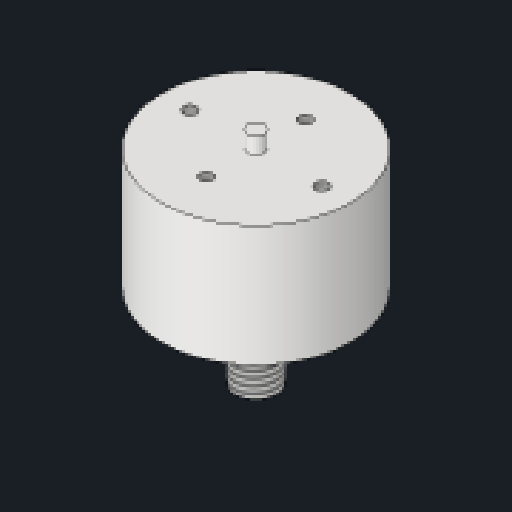
# Autodesk Inventor part: Emax 1806 2280kv
Saved by Autodesk Inventor 2023.2 (Build 272271030, 271C)
## iProperties
Created: 2024-02-18
Part Number: Emax 1806 2280kv
Material: Generic
Document SubType Name: Modeling
Designer: robpl
Density: 1 g/cm^3
Appearance: Default
Author: robpl
Autodesk Inventor part; units mm, degrees
ref_plane "YZ Plane" through (0, 0, 0) normal (1, 0, 0) x (0, 1, 0)
ref_plane "XZ Plane" through (0, 0, 0) normal (0, 1, 0) x (-1, 0, 0)
ref_plane "XY Plane" through (0, 0, 0) normal (0, 0, 1) x (1, 0, 0)
sketch "Sketch1" plane through (0, 0, 0) normal (0, 0, 1) x (1, 0, 0)
  line L0 (0, 0) -> (-11.5, 0)
  line L1 (-11.5, 0) -> (-11.5, -24.7)
  line L2 (-11.5, -24.7) -> (0, -24.7)
  line L3 (0, -24.7) -> (0, 0)
  line L4 (0, -24.7) -> (-2.5, -24.7)
  line L5 (-2.5, -24.7) -> (-2.5, -14.7)
  line L6 (-2.5, -14.7) -> (0, -14.7)
  line L7 (0, -14.7) -> (0, -24.7)
  line L8 (0, 0) -> (-1, 0)
  line L9 (-1, 0) -> (-1, 2)
  line L10 (-1, 2) -> (0, 2)
  line L11 (0, 2) -> (0, 0)
  line L12 (0, -14.7) -> (-11.5, -14.7)
  line L13 (-11.5, -14.7) -> (-11.5, 0)
  line L14 (-11.5, 0) -> (0, 0)
  line L15 (0, 0) -> (0, -14.7)
  dimension "d0" = 11.5
  dimension "d1" = 24.7
  dimension "d2" = 2.5
  dimension "d3" = 10
  dimension "d4" = 1
  dimension "d5" = 2
  constraints: 32 end point, 8 parallel, 4 horizontal, 4 perpendicular
  measures "d0" distance of L2.end L1.end
  measures "d1" distance of L1.end L0.end
  measures "d2" distance of L5.end L6.end
  measures "d3" distance of L4.end L5.end
  measures "d4" distance of L9.end L10.end
  measures "d5" distance of L8.end L9.end
revolve "Revolution1" add sketch "Sketch1" angle 360 about axis through (0, 0, 0) along (0, -1, 0) contours L3 L6 L12 L1 L0 | L0 L9 L10 L11 | L3 L2 L5 L6
thread "Thread1" size "M5x0.8" class "6g" standard "ANSI Metric M Profile" length 7 offset 3
sketch "Sketch2" plane through (0, 0, 0) normal (0, 1, 0) x (1, 0, 0)
  point P0 (0, 0)
  point P1 (8, 0)
  point P2 (-8, 0)
  point P3 (0, -6)
  point P4 (0, 6)
  dimension "d9" = 6
  dimension "d10" = 6
  dimension "d11" = 8
  dimension "d12" = 8
  constraints: 2 horizontal alignment, 2 vertical alignment
  measures "d9" distance of point (0, 0) point (0, 6)
  measures "d10" distance of point (0, -6) point (0, 0)
  measures "d11" distance of point (-8, 0) point (0, 0)
  measures "d12" distance of point (8, 0) point (0, 0)
hole "Hole1" at (8, 0, 0) at (-8, 0, 0) at (0, 0, 6) at (0, 0, -6) direction (0, -1, 0) diameter 1.567 depth 6.3 tip angle 118 thread size "M2x0.4" class "6H" standard "ISO Metric profile"
equation "\"d10\" = d9"
equation "\"d12\" = d11"
body "Solid1"
